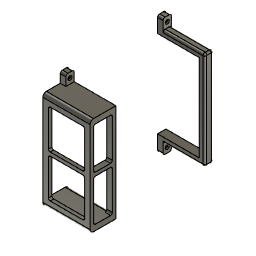
glove-dispenser (Autodesk Fusion 360 design; units mm, degrees)
Autodesk Fusion 360 part; units mm, degrees
sketch "Sketch1" plane through (0, 0, 0) normal (0, 1, 0) x (1, 0, 0)
  line L0 (0, 0) -> (0, -70.5)
  line L1 (0, -70.5) -> (-68, -70.5)
  line L2 (-68, -70.5) -> (-68, -62.5)
  line L3 (-68, -62.5) -> (-8, -62.5)
  line L4 (-8, -62.5) -> (-8, 0)
  line L5 (-8, 0) -> (0, 0) construction
  line L6 (0, 70.5) -> (-68, 70.5)
  line L7 (0, 0) -> (0, 70.5)
  line L8 (-68, 62.5) -> (-8, 62.5)
  line L9 (-8, 62.5) -> (-8, 0)
  line L10 (-68, 70.5) -> (-68, 62.5)
  dimension "d3" = 60
  dimension "d5" = 62.5
  dimension "d6" = 8
  dimension "d7" = 8
  constraint coincident L0.start L5.end
  constraint vertical L0
  constraint perpendicular L0 L1
  constraint perpendicular L1 L2
  constraint perpendicular L2 L3
  constraint perpendicular L3 L4
  constraint perpendicular L0 L5
  constraint symmetric L0.start L5 L7.start
  constraint symmetric L0.end L5 L6.start
  constraint symmetric L1.end L5 L6.end
  constraint symmetric L2.end L5 L8.start
  constraint symmetric L3.end L5 L8.end
  constraint symmetric L4.end L5 L9.end
  measures "d3" distance of L2.end L3.end
  measures "d5" distance of L3.end L4.end
  measures "d6" distance of L4.end L0.start
  measures "d7" distance of L1.end L2.end
extrude "Extrude1" add sketch "Sketch1" along normal blind 12 makes body 1
sketch "Sketch2" plane through (0, 0, 0) normal (1, 0, 0) x (0, 1, 0)
  line L0 (0, 70.5) -> (0, -70.5)
  line L1 (0, -70.5) -> (12, -70.5)
  line L2 (12, -70.5) -> (12, 70.5)
  line L3 (12, 70.5) -> (0, 70.5)
  line L4 (0, 70.5) -> (0, -70.5)
  line L5 (0, 70.5) -> (12, 70.5)
  line L6 (12, 70.5) -> (12, -70.5)
  line L7 (0, -70.5) -> (12, -70.5)
  line L8 (12, 0) -> (0, 0) construction
  line L9 (0, 70.5) -> (0, 85.5)
  line L10 (12, 70.5) -> (12, 85.5)
  line L11 (12, 85.5) -> (0, 85.5)
  line L12 (6, 85.5) -> (6, 70.5) construction
  line L13 (0, 78) -> (12, 78) construction
  circle A0 centre (6, 78) radius 1.5
  circle A1 centre (6, 78) radius 2.875
  circle A2 centre (6, -78) radius 2.875
  circle A3 centre (6, -78) radius 1.5
  line L14 (12, -70.5) -> (12, -85.5)
  line L15 (12, -85.5) -> (0, -85.5)
  line L16 (0, -70.5) -> (0, -85.5)
  dimension "d10" = 15
  dimension "d11" = 3
  dimension "d12" = 5.75
  constraint midpoint L6 L8.start
  constraint coincident L8.end origin
  constraint coincident L0.start L3.end
  constraint perpendicular L5 L9
  constraint coincident L2.end L3.start
  constraint perpendicular L5 L10
  constraint perpendicular L10 L11
  constraint midpoint L11 L12.start
  constraint midpoint L5 L12.end
  constraint midpoint L9 L13.start
  constraint midpoint L10 L13.end
  constraint midpoint L13 A0.centre
  constraint concentric A0 A1
  constraint symmetric L8 L0.start L0.end
  constraint symmetric L8 L9.end L15.end
  constraint symmetric L8 L2.end L1.end
  constraint symmetric L8 L10.end L14.end
  constraint symmetric L8 A0 A3
  constraint symmetric L8 A1 A2
  measures "d10" distance of L0.start L9.end
  measures "d11" diameter of A0
  measures "d12" diameter of A1
extrude "Extrude2" add sketch "Sketch2" along normal blind 8 from surface at -68 contours L3 L5 L9 L10 L11 | L1 L7 L14 L15 L16 | A1 | A2 bodies 1
extrude "Extrude3" cut sketch "Sketch2" against normal blind 2.25 from surface at -60 contours A1 | A2 bodies 1
fillet "Fillet2" radius 3 2 edges at (-64, 0, 85.5) (-64, 12, 85.5) on bodies 1
fillet "Fillet4" radius 3 2 edges at (-64, 12, -85.5) (-64, 0, -85.5) on bodies 1
copy_body "CopyPasteBodies1" bodies 1 makes body 2
fillet "Fillet1" radius 3 2 edges at (-30, 12, 70.5) (-30, 0, 70.5) on bodies 1
fillet "Fillet3" radius 3 2 edges at (-30, 12, -70.5) (-30, 0, -70.5) on bodies 1
fillet "Fillet5" radius 2.5 8 edges at (0, 6, -70.5) (0, 0.8787, -69.6213) (0, 0, 0) (0, 0.8787, 69.6213) (0, 6, 70.5) (0, 11.1213, 69.6213) (0, 12, 0) (0, 11.1213, -69.6213) on bodies 1
sketch "Sketch3" plane through (0, 0, 0) normal (1, 0, 0) x (0, 1, 0)
  line L0 (0, 70.5) -> (0, -70.5)
  line L1 (0, 70.5) -> (12, 70.5)
  line L2 (0, -70.5) -> (12, -70.5)
  line L3 (12, 70.5) -> (12, -70.5)
  line L4 (0, 70.5) -> (-25, 70.5)
  line L5 (-25, 70.5) -> (-25, -70.5)
  line L6 (-25, -70.5) -> (0, -70.5)
  dimension "d29" = 25
  constraint coincident L0.start L1.start
  constraint perpendicular L0 L4
  constraint perpendicular L4 L5
  constraint coincident L0.end L2.start
  constraint perpendicular L0 L6
  measures "d29" distance of L0.start L4.end
extrude "Extrude4" add sketch "Sketch3" against normal up to surface (68 mm away) contours L0 L4 L5 L6 bodies 2
sketch "Sketch4" plane through (0, 0, 0) normal (0, 1, 0) x (-1, 0, 0)
  line L0 (68, 62.5) -> (8, 62.5)
  line L1 (8, 62.5) -> (8, -62.5)
  line L2 (8, -62.5) -> (68, -62.5)
  line L3 (68, -62.5) -> (68, 62.5)
  line L4 (60, 62.5) -> (60, -62.5)
  line L5 (60, 70.5) -> (60, 82.5)
  constraint coincident L0 L4.start
  constraint coincident L2 L4.end
  constraint perpendicular L2 L4
  constraint collinear L4 L5
extrude "Extrude5" cut sketch "Sketch4" against normal blind 20 contours L0 L1 L2 L4 bodies 2
extrude "Extrude6" cut 1 faces at (-65.3333, 0, -20.8333) along direction (0, -1, 0) up to surface (20 mm away) on bodies 2 bodies 2
fillet "Fillet6" radius 5 2 edges at (-34, -25, 70.5) (-34, -25, -70.5) on bodies 2
sketch "Sketch5" plane through (0, -20, 0) normal (0, 1, 0) x (-1, 0, 0)
  line L0 (8, 62.5) -> (8, -62.5)
  line L1 (8, -62.5) -> (68, -62.5)
  line L2 (68, -62.5) -> (68, 62.5)
  line L3 (68, 62.5) -> (8, 62.5)
  line L4 (8, 58.5) -> (60, 58.5)
  line L5 (60, 58.5) -> (60, -58.5)
  line L6 (60, -58.5) -> (8, -58.5)
  line L7 (8, -58.5) -> (8, 58.5)
  line L8 (60, 0) -> (8, 0) construction
  line L9 (8, 2.5) -> (60, 2.5)
  line L10 (8, -2.5) -> (60, -2.5)
  dimension "d38" = 4
  dimension "d39" = 4
  dimension "d40" = 8
  dimension "d53" = 2.5
  constraint horizontal L4
  constraint vertical L5
  constraint horizontal L6
  constraint vertical L7
  constraint collinear L0 L7
  constraint midpoint L5 L8.start
  constraint midpoint L7 L8.end
  constraint coincident L7 L9.start
  constraint coincident L0 L9.start
  constraint coincident L5 L9.end
  constraint perpendicular L5 L9
  constraint symmetric L8 L9.start L10.start
  constraint symmetric L8 L9.end L10.end
  measures "d38" distance of L3 L4
  measures "d39" distance of L1 L6
  measures "d40" distance of L2 L5
  measures "d53" distance of L8 L9
extrude "Extrude7" cut sketch "Sketch5" against normal up to surface (5 mm away) contours L0 L4 L5 L7 L9 | L0 L5 L6 L7 L10 bodies 2
fillet "Fillet7" radius 2.5 4 edges at (-60, -22.5, -58.5) (-8, -22.5, -58.5) (-8, -22.5, 58.5) (-60, -22.5, 58.5) on bodies 2
sketch "Sketch7" plane through (0, 0, 0) normal (1, 0, 0) x (0, 1, 0)
  arc A0 (-25, -65.5) -> (-20, -70.5) centre (-20, -65.5) ccw
  line L0 (-20, -70.5) -> (12, -70.5)
  line L1 (12, -70.5) -> (12, 70.5)
  line L2 (12, 70.5) -> (-20, 70.5)
  arc A1 (-20, 70.5) -> (-25, 65.5) centre (-20, 65.5) ccw
  line L3 (-25, 65.5) -> (-25, -65.5)
  line L4 (-20, 62.5) -> (7, 62.5)
  line L5 (7, 62.5) -> (7, -62.5)
  line L6 (7, -62.5) -> (-20, -62.5)
  line L7 (-20, -62.5) -> (-20, 62.5)
  line L8 (-20, 0) -> (7, 0) construction
  line L9 (-20, 2.5) -> (7, 2.5)
  line L10 (-20, -2.5) -> (7, -2.5)
  dimension "d45" = 8
  dimension "d46" = 5
  dimension "d47" = 5
  dimension "d48" = 8
  dimension "d51" = 2.5
  constraint horizontal L4
  constraint vertical L5
  constraint horizontal L6
  constraint vertical L7
  constraint midpoint L7 L8.start
  constraint midpoint L5 L8.end
  constraint coincident L7 L9.start
  constraint coincident L5 L9.end
  constraint perpendicular L5 L9
  constraint symmetric L8 L9.start L10.start
  constraint symmetric L8 L9.end L10.end
  measures "d45" distance of L2 L4
  measures "d46" distance of L1 L5
  measures "d47" distance of L3 L7
  measures "d48" distance of L0 L6
  measures "d51" distance of L8 L9
extrude "Extrude8" cut sketch "Sketch7" against normal blind 15 contours L4 L5 L7 L9 | L5 L6 L7 L10 bodies 2
fillet "Fillet8" radius 2.5 8 edges at (-4, 7, 62.5) (-34, -20, 62.5) (-4, -20, -2.5) (-4, 7, 2.5) (-4, -20, 2.5) (-4, 7, -2.5) (-34, -20, -62.5) (-4, 7, -62.5) on bodies 2
fillet "Fillet9" radius 5 2 edges at (-38, 12, 62.5) (-38, 12, -62.5) on bodies 2
fillet "Fillet10" radius 2.5 4 edges at (-8, -22.5, 2.5) (-60, -22.5, 2.5) (-60, -22.5, -2.5) (-8, -22.5, -2.5) on bodies 2
move_body "Move1" bodies 1 to x (1, 0, 0) y (0, 1, 0) z (0, 0, 1) at (0, 140, 0)
equation "d5 = ( 125 / 2 ) * 1 mm"
named bodies: "dispenser-top", "dispenser-right", "dispenser-bottom"
